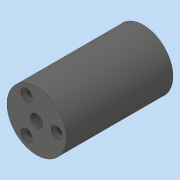
# Autodesk Inventor part: FixedCylinderWireStorage
Saved by Autodesk Inventor 2017 (Build 210142000, 142)
## iProperties
Created: 2016-11-14
Part Number: FixedCylinderWireStorage
Material: ABS Plastic
Document SubType Name: Modeling
Designer: techn
Density: 1.06 g/cm^3
Appearance: Gray
Author: techn
Autodesk Inventor part; units mm, degrees
ref_plane "YZ Plane" through (0, 0, 0) normal (1, 0, 0) x (0, 1, 0)
ref_plane "XZ Plane" through (0, 0, 0) normal (0, 1, 0) x (-1, 0, 0)
ref_plane "XY Plane" through (0, 0, 0) normal (0, 0, 1) x (1, 0, 0)
sketch "Sketch1" plane through (0, 0, 0) normal (0, 0, 1) x (1, 0, 0)
  circle A0 centre (0, 0) radius 15.875
  circle A1 centre (0, 0) radius 13.97
  dimension "d0" = 31.75
  dimension "d1" = 27.94
  constraints: 2 centre point, 2 coincident
  measures "d0" diameter of A0
  measures "d1" diameter of A1
extrude "Extrusion1" add sketch "Sketch1" along normal blind 57.15
sketch "Sketch2" plane through (0, 0, 0) normal (0, 0, -1) x (-1, 0, 0)
  line L0 (0, 0) -> (0, 12.7)
  circle A0 centre (0, 12.7) radius 1.27
  circle A1 centre (0, 12.7) radius 3.175
  circle A2 centre (-10.9985, 6.35) radius 3.175
  circle A3 centre (-10.9985, 6.35) radius 1.27
  circle A4 centre (-10.9985, -6.35) radius 3.175
  circle A5 centre (-10.9985, -6.35) radius 1.27
  circle A6 centre (0, -12.7) radius 3.175
  circle A7 centre (0, -12.7) radius 1.27
  circle A8 centre (10.9985, -6.35) radius 3.175
  circle A9 centre (10.9985, -6.35) radius 1.27
  circle A10 centre (10.9985, 6.35) radius 3.175
  circle A11 centre (10.9985, 6.35) radius 1.27
  dimension "d4" = 12.7
  dimension "d5" = 2.54
  dimension "d6" = 6.35
  dimension "d9" = 360
  constraints: 12 centre point, 7 coincident, 2 end point, 1 vertical, 25 other
  measures "d4" distance of L0.start L0.end
  measures "d5" diameter of A0
  measures "d6" diameter of A1
extrude "Extrusion2" add sketch "Sketch2" against normal up to surface (57.15 mm away) contours A0 | A1 | A2 | A3 | A4 | A5 | A6 | A7 | A8 | A9 | A10 | A11
extrude "Extrusion3" cut sketch "Sketch2" against normal blind 19.05 contours A0 | A3 | A5 | A7 | A9 | A11
sketch "Sketch3" plane through (0, 0, 57.15) normal (0, 0, 1) x (1, 0, 0)
  circle A0 centre (0, 0) radius 3.3655
  circle A1 centre (0, 0) radius 13.97 projected
  dimension "d15" = 6.731
  constraints: 1 centre point, 1 coincident
  measures "d15" diameter of A0
extrude "Extrusion4" add sketch "Sketch3" against normal blind 3.175
fillet "Fillet1" radius 3.175 12 edges at (3.0337, 13.6366, 26.9875) (-3.0337, 13.6366, 26.9875) (10.2928, 9.4456, 26.9875) (13.3265, 4.191, 26.9875) (13.3265, -4.191, 26.9875) (10.2928, -9.4456, 26.9875) (3.0337, -13.6366, 26.9875) (-3.0337, -13.6366, 26.9875) (-10.2928, -9.4456, 26.9875) (-13.3265, -4.191, 26.9875) (-13.3265, 4.191, 26.9875) (-10.2928, 9.4456, 26.9875)
sketch "Sketch7" plane through (0, 0, 57.15) normal (0, 0, 1) x (1, 0, 0)
  circle A0 centre (-5.3975, 9.3487) radius 3.048
  line L0 (0, 0) -> (0, 13.3395) construction
  circle A1 centre (-5.3975, 9.3487) radius 1.5875
  circle A2 centre (-5.3975, -9.3487) radius 3.048
  circle A3 centre (-5.3975, -9.3487) radius 1.5875
  circle A4 centre (10.795, 0) radius 3.048
  circle A5 centre (10.795, 0) radius 1.5875
  dimension "d23" = 6.096
  dimension "d24" = 10.795
  dimension "d25" = 30
  dimension "d26" = 3.175
  dimension "d29" = 360
  constraints: 6 centre point, 3 coincident, 2 end point, 1 vertical, 13 other
  measures "d23" diameter of A0
  measures "d24" distance of L0.start A0.centre
  measures "d26" diameter of A1
extrude "Extrusion6" cut sketch "Sketch7" against normal blind 0.635 contours A0 | A1 | A2 | A3 | A4 | A5
extrude "Extrusion7" cut sketch "Sketch7" against normal through all contours A1 | A3 | A5
chamfer "Chamfer1" distance 1.4605 angle 45 3 edges at (-6.985, -9.3487, 56.515) (-6.985, 9.3487, 56.515) (9.2075, 0, 56.515)
body "Solid1"
